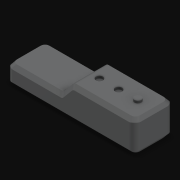
# Autodesk Inventor part: V5_Simple_rADIO
Saved by Autodesk Inventor 2021 (Build 250183000, 183)
## iProperties
Created: 2020-06-10
Part Number: V5_Simple_rADIO
Material: Generic
Document SubType Name: Modeling
Designer: Charlie Grier
Density: 1 g/cm^3
Appearance: Default
Author: Charlie Grier
Autodesk Inventor part; units mm, degrees
ref_plane "YZ Plane" through (0, 0, 0) normal (1, 0, 0) x (0, 1, 0)
ref_plane "XZ Plane" through (0, 0, 0) normal (0, 1, 0) x (-1, 0, 0)
ref_plane "XY Plane" through (0, 0, 0) normal (0, 0, 1) x (1, 0, 0)
sketch "Sketch1" plane through (0, 0, 0) normal (0, 0, 1) x (1, 0, 0)
  line L0 (-42.2529, -10.5029) -> (42.2529, -10.5029)
  line L1 (42.2529, -10.5029) -> (42.2529, 10.5029)
  line L2 (42.2529, 10.5029) -> (-42.2529, 10.5029)
  line L3 (-42.2529, 10.5029) -> (-42.2529, -10.5029)
  line L4 (-42.2529, -10.5029) -> (42.2529, 10.5029) construction
  line L5 (42.2529, -10.5029) -> (-42.2529, 10.5029) construction
  point P0 (0, 0)
  dimension "d0" = 84.5058
  dimension "d1" = 21.0058
  constraints: 12 end point, 2 midpoint, 2 parallel, 1 horizontal, 1 perpendicular
  measures "d0" distance between parallel lines of L1 L3
  measures "d1" distance between parallel lines of L0 L2
extrude "Extrusion1" add sketch "Sketch1" along normal blind 25.4
sketch "Sketch2" plane through (0, 0, 25.4) normal (0, 0, 1) x (1, 0, 0)
  line L0 (42.2529, -10.5029) -> (42.2529, 10.5029) projected
  line L1 (-42.2529, -10.5029) -> (42.2529, -10.5029) projected
  line L2 (42.2529, 10.5029) -> (-42.2529, 10.5029) projected
  line L3 (-42.2529, 10.5029) -> (-42.2529, -10.5029) projected
  line L4 (-42.2529, 1.9939) -> (-6.7246, 1.9939)
  line L5 (-6.7246, 1.9939) -> (0.4152, 10.5029)
  line L6 (0.4152, 10.5029) -> (-42.2529, 10.5029)
  line L7 (-42.2529, 1.9939) -> (-42.2529, 10.5029)
  point P0 (0, 0)
  dimension "d5" = 48.9776
  dimension "d6" = 12.4968
  dimension "d7" = 0
  dimension "d10" = 130
  constraints: 8 end point, 1 horizontal, 1 point on line
  measures "d5" distance from line of L0 L4.end
  measures "d6" distance from line of L1 L4.end
  measures "d7" distance from line of L2 L5.end
  measures "d10" angle of L5 L4
extrude "Extrusion2" cut sketch "Sketch2" against normal through all contours L5 L4 L3 L2
chamfer "Chamfer1" distance 1.9558 distance2 2.4384 1 edges at (21.3341, 10.5029, 0) measured on face at (28.307, 10.5029, 16.9333)
chamfer "Chamfer2" distance 2.4384 distance2 1.4986 1 edges at (42.2529, 10.5029, 13.6779) measured on face at (42.2529, 3.501, 17.5853)
chamfer "Chamfer3" distance 2.4384 distance2 1.9558 1 edges at (20.5848, 10.5029, 25.4) measured on face at (-2.2415, -6.3373, 25.4)
chamfer "Chamfer4" distance 2.4384 distance2 1.9558 1 edges at (-4.1777, 5.0292, 25.4) measured on face at (-2.2415, -6.3373, 25.4)
chamfer "Chamfer5" distance 2.4384 distance2 1.9558 1 edges at (-24.4888, 1.9939, 25.4) measured on face at (-1.1805, -6.3373, 25.4)
chamfer "Chamfer6" distance 2.4384 distance2 1.9558 1 edges at (-4.1777, 5.0292, 0) measured on face at (-2.2415, -6.3373, 0)
chamfer "Chamfer7" distance 2.4384 distance2 1.9558 1 edges at (-24.4888, 1.9939, 0) measured on face at (-1.1805, -6.3373, 0)
chamfer "Chamfer8" distance 2.5146 distance2 2.5908 1 edges at (0, -10.5029, 25.4) measured on face at (-14.0843, -10.5029, 8.4667)
chamfer "Chamfer9" distance 2.5146 distance2 2.5908 1 edges at (0, -10.5029, 0) measured on face at (-14.0843, -10.5029, 7.6285)
chamfer "Chamfer10" distance 1.8796 distance2 2.5908 1 edges at (-42.2529, -10.5029, 12.7) measured on face at (-14.0843, -10.5029, 9.3049)
chamfer "Chamfer11" distance 1.8796 distance2 2.5908 1 edges at (42.2529, -10.5029, 12.7) measured on face at (-12.8312, -10.5029, 16.0951)
chamfer "Chamfer12" distance 1.778 distance2 2.5908 1 edges at (-42.2529, 1.9939, 12.7) measured on face at (-30.4101, 1.9939, 9.1186)
fillet "Fillet1" radius 2.4892 2 edges at (-6.7246, 1.9939, 12.7) (0.4152, 10.5029, 12.7)
fillet "Fillet2" radius 3.7592 16 edges at (-42.2529, -4.2545, 25.4) (42.2529, 0.0762, 25.4) (42.2529, 0.0762, 0) (-42.2529, -4.2545, 0) (-41.3116, 0.7747, 24.4221) (-41.3116, 0.7747, 0.9779) (-41.3131, -9.2075, 1.2573) (-41.3131, -9.2075, 24.1427) (41.3131, -9.2075, 24.1427) (41.3131, -9.2075, 1.2573) (41.5036, 9.2837, 24.4221) (41.5036, 9.2837, 0.9779) (-6.2105, 0.8913, 24.3286) (1.0381, 9.1671, 24.5156) (-6.2105, 0.8913, 1.0714) (1.0381, 9.1671, 0.8844)
sketch "Sketch3" plane through (1.576, 10.5029, 23.4442) normal (0, 1, 0) x (1, 0, 0)
  circle A0 centre (30.0597, 10.7442) radius 2.286
  line L0 (40.6769, 1.8034) -> (40.6769, 19.685) projected
  line L1 (1.0731, -1.9558) -> (36.9177, -1.9558) projected
  circle A1 centre (17.3597, 10.7442) radius 2.286
  circle A2 centre (4.6597, 10.7442) radius 2.286
  point P0 (-1.576, 23.4442)
  dimension "HoleSize" = 4.572
  dimension "d50" = 10.6172
  dimension "d51" = 12.7
  dimension "d52" = 4.572
  dimension "d53" = 4.572
  dimension "d54" = 12.7
  dimension "d55" = 12.7
  dimension "d56" = 12.7
  dimension "d57" = 12.7
  constraints: 3 centre point
  measures "HoleSize" diameter of A0
  measures "d50" distance from line of L0 A0.centre
  measures "d51" distance from line of L1 A0.centre
  measures "d52" diameter of A1
  measures "d53" diameter of A2
  measures "d54" distance of A1.centre A0.centre
  measures "d55" distance of A2.centre A1.centre
  measures "d56" distance from line of L1 A1.centre
  measures "d57" distance from line of L1 A2.centre
extrude "Extrusion3" cut sketch "Sketch3" against normal blind 1.5875 contours A1 | A2
sketch "Sketch6" plane through (1.576, 10.5029, 23.4442) normal (0, 1, 0) x (1, 0, 0)
  circle A0 centre (30.0597, 10.7442) radius 2.286
  circle A1 centre (17.3597, 10.7442) radius 2.286 projected
  line L0 (1.0731, -1.9558) -> (36.9177, -1.9558) projected
  point P0 (-1.576, 23.4442)
  dimension "d76" = 4.572
  dimension "d77" = 12.7
  dimension "d78" = 12.7
  constraints: 1 centre point
  measures "d76" diameter of A0
  measures "d77" distance of A1.centre A0.centre
  measures "d78" distance from line of L0 A0.centre
extrude "Extrusion4" add sketch "Sketch6" along normal blind 1.5875 contours A0
equation "\"d52\" = HoleSize"
equation "\"d53\" = HoleSize"
equation "\"d76\" = HoleSize"
body "Solid1"
